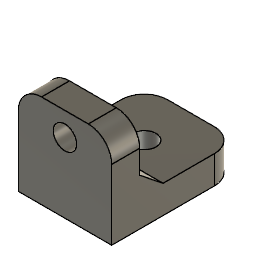
bracket (Autodesk Fusion 360 design; units mm, degrees)
Autodesk Fusion 360 part; units mm, degrees
sketch "Sketch1" plane through (0, 0, 0) normal (0, 0, 1) x (1, 0, 0)
  line L0 (10, 13.5) -> (-10, 13.5)
  line L1 (-10, 13.5) -> (-10, -13.5)
  line L2 (-10, -13.5) -> (10, -13.5)
  line L3 (10, -13.5) -> (10, 13.5)
  line L4 (10, 13.5) -> (-10, -13.5) construction
  line L5 (-10, 13.5) -> (10, -13.5) construction
  circle A0 centre (0, 3.5) radius 2.5
  line L6 (-10, -13.5) -> (10, -13.5)
  line L7 (10, -13.5) -> (10, -7.5)
  line L8 (10, -7.5) -> (-10, -7.5)
  line L9 (-10, -7.5) -> (-10, -13.5)
  dimension "d1" = 20
  dimension "d2" = 27
  dimension "d3" = 5
  dimension "d4" = 10
  dimension "d5" = 6
  constraint horizontal L0
  constraint perpendicular L0 L1
  constraint parallel L0 L2
  constraint parallel L1 L3
  constraint coincident L4 origin
  constraint coincident L5 origin
  constraint vertical origin A0.centre
  constraint horizontal L6
  constraint vertical L7
  constraint horizontal L8
  constraint vertical L9
  constraint coincident L3 L7.end
  measures "d1" distance of L1.end L2.end
  measures "d2" distance of L0.end L1.end
  measures "d3" diameter of A0
  measures "d4" distance of L0 A0.centre
  measures "d5" distance of L1.end L8.end
extrude "Extrude1" add sketch "Sketch1" along normal blind 6 contours L0 L1 L3 L8
extrude "Extrude2" add sketch "Sketch1" along normal blind 20 contours L1 L2 L3 L6 L7 L8 L9
sketch "Sketch2" plane through (0, -13.5, 0) normal (0, -1, 0) x (1, 0, 0)
  line L0 (-10, 0) -> (10, 0)
  line L1 (10, 0) -> (10, 20)
  line L2 (10, 20) -> (-10, 20)
  line L3 (-10, 20) -> (-10, 0)
  circle A0 centre (0, 15) radius 2.5
  dimension "d10" = 5
  dimension "d11" = 15
  constraint vertical origin A0.centre
  measures "d10" diameter of A0
  measures "d11" distance of origin A0.centre
extrude "Extrude3" cut sketch "Sketch2" against normal blind 90 contours A0
chamfer "Chamfer1" distance 5 distance2 4 1 edges at (0, -7.5, 6) measured on face at (-0.0623, -4.6643, 6)
fillet "Fillet1" radius 5 4 edges at (10, 13.5, 3) (-10, 13.5, 3) (-10, -10.5, 20) (10, -10.5, 20)
